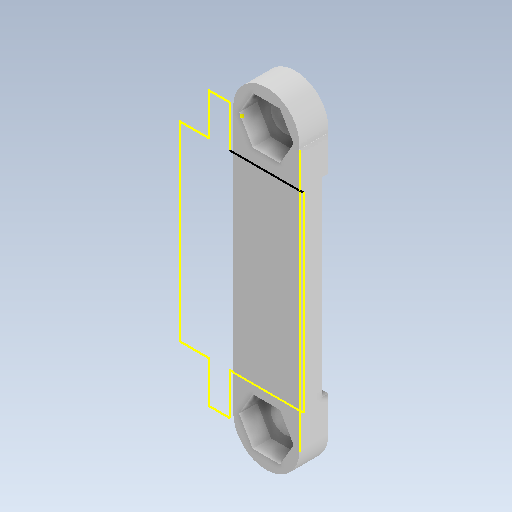
# Autodesk Inventor part: крышка_держалка_серво_брови
Saved by Autodesk Inventor 2020 (Build 240168000, 168)
## iProperties
Created: 2022-03-05
Part Number: крышка_держалка_серво_брови
Material: Типовые
Document SubType Name: Modeling
Designer: Администратор
Density: 1 g/cm^3
Appearance: По умолчанию
Author: Администратор
Autodesk Inventor part; units mm, degrees
ref_plane "YZ Plane" through (0, 0, 0) normal (1, 0, 0) x (0, 1, 0)
ref_plane "XZ Plane" through (0, 0, 0) normal (0, 1, 0) x (-1, 0, 0)
ref_plane "XY Plane" through (0, 0, 0) normal (0, 0, 1) x (1, 0, 0)
sketch "Эскиз1" plane through (0, 0, 0) normal (0, 0, 1) x (1, 0, 0)
  line L0 (-7.5, -27.25) -> (-4, -27.25) projected
  line L1 (-4, -27.25) -> (-4, -32.25) projected
  line L2 (-4, -32.25) -> (-1.5, -32.25) projected
  line L3 (-1.5, -32.25) -> (-1.5, -27.25) projected
  line L4 (-1.5, -27.25) -> (7.5, -27.25) projected
  line L5 (7.5, -4.25) -> (7.5, -27.25) projected
  line L6 (7.5, -4.25) -> (-1.5, -4.25) projected
  line L7 (-1.5, -4.25) -> (-1.5, 0.75) projected
  line L8 (-1.5, 0.75) -> (-4, 0.75) projected
  line L9 (-4, 0.75) -> (-4, -4.25) projected
  line L10 (-4, -4.25) -> (-7.5, -4.25) projected
  line L11 (-7.5, -27.25) -> (-7.5, -4.25) projected
  line L12 (7.5, 0) -> (6.75, 0)
  line L13 (7, 0) -> (7, -31.5)
  line L14 (-1, 0) -> (3, 0)
  arc A0 (-1, -31.5) -> (7, -31.5) centre (3, -31.5) ccw
  line L15 (-1, 0) -> (-1, -31.5)
  line L16 (7, 0) -> (7, 0.5)
  line L17 (-1, 0) -> (-1, 0.5)
  arc A1 (6.9686, 0) -> (-0.9686, 0) centre (3, 0.5) ccw
  line L18 (-1, 0) -> (-0.9686, 0)
  line L19 (6.9686, 0) -> (7, 0)
  point P0 (0, 0)
  point P1 (6.9686, 0)
  dimension "d15" = 4
  dimension "d25" = 31.5
  dimension "d26" = 0.5
  dimension "d27" = 0.5
  constraints: 16 end point, 5 point on circle, 3 vertical, 2 centre point, 2 point on line, 1 horizontal, 1 parallel
  measures "d15" distance of L14.start L14.end
  measures "d25" distance of L13.start L13.end
  measures "d26" distance of L13.start L16.end
  measures "d27" distance of L14.start L17.end
extrude "Выдавливание1" add sketch "Эскиз1" along normal blind 3.5 contours L15 L6 L13 L4 | L4 L13 A0 L15 | L15 L14 A1 L12 L13 L6
sketch "Эскиз2" plane through (0, 0, 3.5) normal (0, 0, 1) x (1, 0, 0)
  line L0 (-7.5, -27.25) -> (-4, -27.25) projected
  line L1 (-4, -27.25) -> (-4, -32.25) projected
  line L2 (-4, -32.25) -> (-1.5, -32.25) projected
  line L3 (-1.5, -32.25) -> (-1.5, -27.25) projected
  line L4 (-1.5, -27.25) -> (7.5, -27.25) projected
  line L5 (7.5, -4.25) -> (7.5, -27.25) projected
  line L6 (7.5, -4.25) -> (-1.5, -4.25) projected
  line L7 (-1.5, -4.25) -> (-1.5, 0.75) projected
  line L8 (-1.5, 0.75) -> (-4, 0.75) projected
  line L9 (-4, 0.75) -> (-4, -4.25) projected
  line L10 (-4, -4.25) -> (-7.5, -4.25) projected
  line L11 (-7.5, -27.25) -> (-7.5, -4.25) projected
  line L12 (-1.5, -4.25) -> (7.5, -4.25)
  line L13 (7, -31.5) -> (7, 0) projected
  point P0 (0, 0)
  constraints: 2 end point, 1 perpendicular
sketch "Эскиз4" plane through (0, 0, 0) normal (0, 0, 1) x (1, 0, 0)
  line L0 (-0.2909, -31.25) -> (1.3546, -28.4) projected
  line L1 (1.3546, -28.4) -> (4.6454, -28.4) projected
  line L2 (4.6454, -28.4) -> (6.2909, -31.25) projected
  line L3 (6.2909, -31.25) -> (4.6454, -34.1) projected
  line L4 (4.6454, -34.1) -> (1.3546, -34.1) projected
  line L5 (1.3546, -34.1) -> (-0.2909, -31.25) projected
  arc A0 (-1, -31.5) -> (7, -31.5) centre (3, -31.5) ccw projected
  line L6 (-0.2909, 0.25) -> (1.3546, -2.6)
  line L7 (1.3546, -2.6) -> (4.6454, -2.6)
  line L8 (4.6454, -2.6) -> (6.2909, 0.25)
  line L9 (6.2909, 0.25) -> (4.6454, 3.1)
  line L10 (4.6454, 3.1) -> (1.3546, 3.1)
  line L11 (1.3546, 3.1) -> (-0.2909, 0.25)
  circle A1 centre (3, -31.25) radius 1.65
  circle A2 centre (3, 0.25) radius 1.65
  point P0 (0, 0)
  constraints: 12 end point, 2 centre point, 4 other
sketch "Эскиз5" plane through (0, 0, 0) normal (0, 0, 1) x (1, 0, 0)
  circle A0 centre (3, 0.25) radius 1.65 projected
  circle A1 centre (3, -31.25) radius 1.65 projected
  line L0 (-1, 0) -> (-1, -31.5) projected
  arc A2 (-1, -31.5) -> (7, -31.5) centre (3, -31.5) ccw projected
  line L1 (7, -31.5) -> (7, 0) projected
  line L2 (6.2909, -31.25) -> (4.6454, -34.1) projected
  line L3 (4.6454, -34.1) -> (1.3546, -34.1) projected
  line L4 (1.3546, -34.1) -> (-0.2909, -31.25) projected
  line L5 (4.6454, -34.1) -> (1.3546, -34.1) projected
  line L6 (6.2909, -31.25) -> (4.6454, -34.1) projected
  line L7 (4.6454, -28.4) -> (6.2909, -31.25) projected
  line L8 (1.3546, -28.4) -> (4.6454, -28.4) projected
  line L9 (-0.2909, -31.25) -> (1.3546, -28.4) projected
  circle A3 centre (3, -31.25) radius 1.65
  line L10 (3, -15.75) -> (0.5318, -15.75)
  line L11 (7, 0) -> (6.9686, 0) projected
  arc A4 (6.9686, 0) -> (-0.9686, 0) centre (3, 0.5) ccw projected
  line L12 (-0.9686, 0) -> (-1, 0) projected
  point P0 (0, 0)
  dimension "d24" = 3.3
  constraints: 2 end point, 1 centre point, 1 coincident, 1 horizontal
  measures "d24" diameter of A3
extrude "Выдавливание5" cut sketch "Эскиз5" along normal through all contours A0 | A1
sketch "Эскиз6" plane through (0, 0, 0) normal (0, 0, 1) x (1, 0, 0)
  line L0 (7.5, -4.25) -> (-1.5, -4.25) projected
  line L1 (-1.5, -27.25) -> (7.5, -27.25) projected
  line L2 (-1, 0) -> (-1, -31.5) projected
  line L3 (7, -31.5) -> (7, 0) projected
  line L4 (-1, -4.25) -> (7, -4.25)
  line L5 (7, -4.25) -> (7, -27.25)
  line L6 (7, -27.25) -> (-1, -27.25)
  line L7 (-1, -27.25) -> (-1, -4.25)
  point P0 (0, 0)
  point P1 (-1, -27.25)
  constraints: 8 end point, 4 point on line, 2 parallel, 1 horizontal, 1 perpendicular
extrude "Выдавливание6" cut sketch "Эскиз6" along normal blind 0.8
extrude "Выдавливание7" cut sketch "Эскиз4" along normal through all contours L0 L1 L2 L3 L4 L5 | L11 L10 L9 L8 L7 L6 | A1 | A2
sketch "Эскиз7" plane through (0, 0, 3.5) normal (0, 0, 1) x (1, 0, 0)
  line L0 (-0.2909, -31.25) -> (1.3546, -28.4) projected
  line L1 (1.3546, -28.4) -> (4.6454, -28.4) projected
  line L2 (1.3546, -34.1) -> (-0.2909, -31.25) projected
  line L3 (4.6454, -28.4) -> (6.2909, -31.25) projected
  line L4 (6.2909, -31.25) -> (4.6454, -34.1) projected
  line L5 (4.6454, -34.1) -> (1.3546, -34.1) projected
  line L6 (-1, -4.25) -> (-1, -27.25) projected
  line L7 (7, -27.25) -> (7, -4.25) projected
  line L8 (-1, -27.25) -> (-1, -15.5)
  line L9 (-1, 0) -> (-1, -31.5) projected
  line L10 (-1, -15.5) -> (4.3528, -15.5)
  line L11 (-0.2909, 0.25) -> (1.3546, -2.6)
  line L12 (1.3546, -2.6) -> (4.6454, -2.6)
  line L13 (1.3546, 3.1) -> (-0.2909, 0.25)
  line L14 (4.6454, -2.6) -> (6.2909, 0.25)
  line L15 (6.2909, 0.25) -> (4.6454, 3.1)
  line L16 (4.6454, 3.1) -> (1.3546, 3.1)
  point P0 (-1, 0.5)
  dimension "d31" = 11.75
  constraints: 16 end point, 7 symmetric about line, 1 horizontal, 1 point on line
  measures "d31" distance of L6.end L8.end
extrude "Выдавливание8" cut sketch "Эскиз7" against normal blind 2.2
extrude "Выдавливание9" add sketch "Эскиз4" along normal blind 1.3 contours L0 L1 L2 L3 L4 L5 | L11 L10 L9 L8 L7 L6 | A2
sketch "Эскиз8" plane through (0, 0, 1.3) normal (0, 0, 1) x (1, 0, 0)
  circle A0 centre (3, 0.25) radius 1.65 projected
  point P0 (0, 0)
extrude "Выдавливание10" cut sketch "Эскиз8" against normal through all
